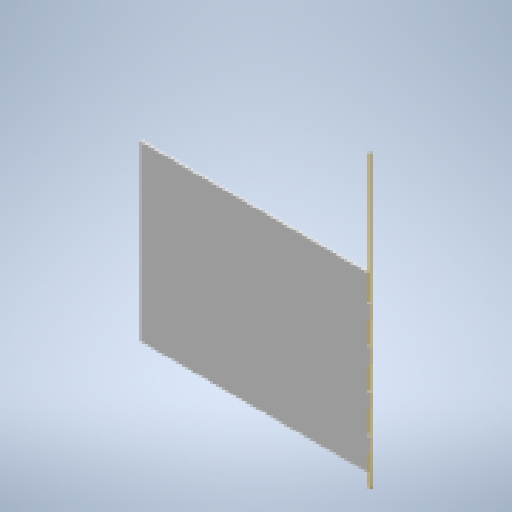
# Autodesk Inventor part: leg 2
Saved by Autodesk Inventor 2023 (Build 270158000, 158)
## iProperties
Created: 2023-09-18
Part Number: leg 2
Material: Polystyrene
Document SubType Name: Modeling
Designer: Nate
Mass: 826.897 g
Surface Area: 3505.13 cm^2
Volume: 809.889 cm^3
Density: 1.021 g/cm^3
Appearance: Smooth - White
Author: Nate
Autodesk Inventor part; units mm, degrees
ref_plane "YZ Plane" through (0, 0, 0) normal (1, 0, 0) x (0, 1, 0)
ref_plane "XZ Plane" through (0, 0, 0) normal (0, 1, 0) x (-1, 0, 0)
ref_plane "XY Plane" through (0, 0, 0) normal (0, 0, 1) x (1, 0, 0)
ref_plane "Work Plane1" through (0, 0, 0) normal (0, 0, 1) x (1, 0, 0)
sketch "Sketch2" plane through (0, 0, 0) normal (0, 0, 1) x (1, 0, 0)
  line L0 (5.0006, 57.6014) -> (-474.9994, 57.6014)
  line L1 (-474.9994, 57.6014) -> (-474.9994, -309.9996)
  line L2 (-474.9994, -309.9996) -> (5.0006, -309.9996)
  line L3 (5.0006, -309.9996) -> (5.0006, 57.6014)
  line L4 (5.0006, -239.9996) -> (0.2381, -239.9996)
  line L5 (0.2381, -239.9996) -> (0.2381, -269.9996)
  line L6 (0.2381, -269.9996) -> (5.0006, -269.9996)
  line L7 (5.0006, -269.9996) -> (5.0006, -239.9996)
  line L8 (5.0006, -159.9996) -> (0.2381, -159.9996)
  line L9 (0.2381, -159.9996) -> (0.2381, -189.9996)
  line L10 (0.2381, -189.9996) -> (5.0006, -189.9996)
  line L11 (5.0006, -189.9996) -> (5.0006, -159.9996)
  line L12 (5.0006, 0.0004) -> (0.2381, 0.0004)
  line L13 (0.2381, 0.0004) -> (0.2381, -29.9996)
  line L14 (0.2381, -29.9996) -> (5.0006, -29.9996)
  line L15 (5.0006, -29.9996) -> (5.0006, 0.0004)
  line L16 (5.0006, -79.9996) -> (0.2381, -79.9996)
  line L17 (0.2381, -79.9996) -> (0.2381, -109.9996)
  line L18 (0.2381, -109.9996) -> (5.0006, -109.9996)
  line L19 (5.0006, -109.9996) -> (5.0006, -79.9996)
  line L20 (5.0006, 57.6014) -> (0.2381, 57.6014)
  line L21 (0.2381, 57.6014) -> (0.2381, -309.9996)
  line L22 (0.2381, -309.9996) -> (5.0006, -309.9996)
  line L23 (5.0006, -309.9996) -> (5.0006, 57.6014)
  line L24 (5.0006, 57.6014) -> (-474.9994, 57.6014)
  line L25 (-474.9994, 57.6014) -> (-474.9994, 54.6014)
  line L26 (-474.9994, 54.6014) -> (5.0006, 54.6014)
  line L27 (5.0006, 54.6014) -> (5.0006, 57.6014)
  line L28 (-474.9994, -309.9996) -> (5.0006, -309.9996)
  line L29 (5.0006, -309.9996) -> (5.0006, -306.9996)
  line L30 (5.0006, -306.9996) -> (-474.9994, -306.9996)
  line L31 (-474.9994, -306.9996) -> (-474.9994, -309.9996)
  line L32 (5.0006, -65.3986) -> (-474.9994, -65.3986)
  line L33 (-474.9994, -65.3986) -> (-474.9994, -75.3986)
  line L34 (-474.9994, -75.3986) -> (5.0006, -75.3986)
  line L35 (5.0006, -75.3986) -> (5.0006, -65.3986)
  line L36 (-474.9994, -65.3986) -> (-235.9994, -65.3986)
  line L37 (-235.9994, -65.3986) -> (-235.9994, -75.3986)
  line L38 (-235.9994, -75.3986) -> (-474.9994, -75.3986)
  line L39 (-474.9994, -75.3986) -> (-474.9994, -65.3986)
  point P0 (0, 0)
  point P1 (0.2381, -306.9996)
  point P2 (0.2381, -239.9996)
  point P3 (0.2381, 54.6014)
  point P4 (-235.9994, -65.3986)
  point P5 (0.2381, -65.3986)
  point P6 (0.2381, -75.3986)
  point P7 (-235.9994, -75.3986)
  dimension "d14" = 480
  dimension "d15" = 367.601
  dimension "d16" = 4.7625
  dimension "d17" = 30
  dimension "d18" = 4.7625
  dimension "d19" = 30
  dimension "d20" = 4.7625
  dimension "d21" = 30
  dimension "d22" = 4.7625
  dimension "d23" = 30
  dimension "d24" = 40
  dimension "d25" = 50
  dimension "d26" = 50
  dimension "d27" = 50
  dimension "d28" = 4.7625
  dimension "d29" = 367.601
  dimension "d30" = 3
  dimension "d31" = 3
  dimension "d34" = 480
  dimension "d35" = 10
  dimension "d36" = 123
  dimension "d37" = 239
  dimension "d38" = 10
  constraints: 80 end point, 20 parallel, 10 horizontal, 10 perpendicular, 4 point on line
  measures "d14" distance of L2.end L1.end
  measures "d15" distance of L1.end L0.end
  measures "d16" distance of L6.end L5.end
  measures "d17" distance of L5.end L4.end
  measures "d18" distance of L11.start L9.end
  measures "d19" distance of L9.end L9.start
  measures "d20" distance of L15.start L13.end
  measures "d21" distance of L13.end L13.start
  measures "d22" distance of L19.start L17.end
  measures "d23" distance of L17.end L17.start
  measures "d24" distance between parallel lines of L2 L6
  measures "d25" distance between parallel lines of L4 L10
  measures "d26" distance between parallel lines of L18 L8
  measures "d27" distance between parallel lines of L14 L16
  measures "d28" distance of L22.end L21.end
  measures "d29" distance of L21.end L20.end
  measures "d30" distance between parallel lines of L26 L0
  measures "d31" distance between parallel lines of L28 L30
  measures "d34" distance of L34.end L33.end
  measures "d35" distance of L33.end L32.end
  measures "d36" distance between parallel lines of L32 L0
  measures "d37" distance of L37.end L38.end
  measures "d38" distance of L36.end L37.end
extrude "Extrusion1" add sketch "Sketch2" along normal blind 4.7625 contours L21 L13 L32 L1 L26 | L3 L14 L13 L12 | L32 L37 L34 L1 | L34 L21 L17 L9 L5 L30 L1 | L3 L18 L17 L16 | L5 L4 L3 L6 | L3 L10 L9 L8
body "Solid1"
